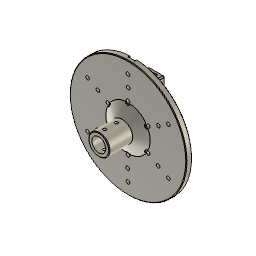
ワインダー量産試作機 (Autodesk Fusion 360 archive; units mm, degrees)
design "ピックアップチャッキ"
Autodesk Fusion 360 part; units mm, degrees
sketch "スケッチ1" plane through (0, 0, 0) normal (0, 0, 1) x (1, 0, 0)
  circle A0 centre (0, 0) radius 50
  dimension "d1" = 100
  constraint coincident A0.centre origin
  measures "d1" diameter of A0
extrude "押し出し1" add sketch "スケッチ1" along normal blind 5 makes body 1
sketch "スケッチ2" plane through (0, 0, 5) normal (0, 0, 1) x (-1, 0, 0)
  circle A0 centre (0, 0) radius 50
  circle A1 centre (0, 0) radius 9
  circle A2 centre (0, 0) radius 6
  dimension "d4" = 18
  dimension "d5" = 12
  constraint concentric A0 A1
  constraint coincident A0.centre A1.centre
  measures "d4" diameter of A1
  measures "d5" diameter of A2
extrude "押し出し2" add sketch "スケッチ2" along normal blind 25 contours A1 bodies 1
sketch "スケッチ3" plane through (0, 0, 0) normal (0, 1, 0) x (1, 0, 0)
  line L0 (9, -5) -> (9, -10)
  line L1 (9, -5) -> (19, -5)
  line L2 (19, -5) -> (9, -10)
  constraint vertical L0
  constraint perpendicular L0 L1
revolve "回転1" add sketch "スケッチ3" angle 360 about axis through (0, 0, 1.75) along (0, 0, 1) bodies 1
chamfer "面取り1" distance 0.5 angle 45 3 edges at (-46.6164, -18.0808, 0) (-46.6164, -18.0808, 5) (8.3909, 3.2545, 30) on bodies 1
sketch "スケッチ4" plane through (0, 0, 0) normal (0, 1, 0) x (1, 0, 0)
  line L0 (0, -30) -> (0, -25)
  line L1 (0, -10) -> (0, -15)
  circle A0 centre (0, -25) radius 1.25
  circle A1 centre (0, -15) radius 1.25
  dimension "d10" = 2.5
  dimension "d11" = 2.5
  constraint vertical L0
  constraint vertical L1
  constraint coincident L0.end A0.centre
  constraint coincident L1.end A1.centre
  measures "d10" diameter of A0
  measures "d11" diameter of A1
extrude "押し出し3" cut sketch "スケッチ4" along normal blind 9 and the other way blind 9 bodies 1
sketch "スケッチ5" plane through (0, 0, 0) normal (0, 0, 1) x (1, 0, 0)
  circle A0 centre (0, -40) radius 1.5
  circle A1 centre (-0.2424, -30) radius 1.5
  circle A2 centre (0, -20) radius 1.5
  point P0 (0, -20)
  point P1 (0, -30)
  point P2 (0, -40)
  dimension "d16" = 3
  dimension "d17" = 3
  dimension "d18" = 3
  constraint coincident P2 A0.centre
  constraint coincident P0 A2.centre
  measures "d16" diameter of A0
  measures "d17" diameter of A1
  measures "d18" diameter of A2
extrude "押し出し4" cut sketch "スケッチ5" along normal blind 6 bodies 1
pattern_circular "C パターン1" count 6 over 360 about axis through (0, 0, 1.75) along (0, 0, 1) of 3 faces at (-1.4095, -39.487, 3.3333) (1.2502, -29.8506, 3.3333) (-1.1427, -19.0283, 3.3333) on bodies 1
sketch "スケッチ6" plane through (0, 0, 0) normal (0, 0, 1) x (1, 0, 0)
  circle A0 centre (0, 0) radius 1.5
  dimension "d23" = 3
  constraint coincident A0.centre origin
  measures "d23" diameter of A0
extrude "押し出し5" cut sketch "スケッチ6" along normal blind 5 bodies 1
sketch "スケッチ7" plane through (0, 0, 5) normal (0, 0, 1) x (-1, 0, 0)
  circle A0 centre (26.1019, 14.7901) radius 1.5
  circle A1 centre (25.8596, -15.2099) radius 1.5
  circle A2 centre (-0.2424, -30) radius 1.5
  circle A3 centre (-26.1019, -14.7901) radius 1.5
  circle A4 centre (-25.8596, 15.2099) radius 1.5
  circle A5 centre (34.641, 20) radius 1.5
  circle A6 centre (34.641, -20) radius 1.5
  circle A7 centre (0, -40) radius 1.5
  circle A8 centre (-34.641, -20) radius 1.5
  circle A9 centre (-34.641, 20) radius 1.5
  arc A10 (16.9721, 8.541) -> (15.8828, 10.4277) centre (17.3205, 10) ccw
  arc A11 (16.9721, -8.541) -> (16.9721, 8.541) centre (0, 0) ccw
  arc A12 (15.8828, -10.4277) -> (16.9721, -8.541) centre (17.3205, -10) ccw
  arc A13 (1.0893, -18.9688) -> (15.8828, -10.4277) centre (0, 0) ccw
  arc A14 (-1.0893, -18.9688) -> (1.0893, -18.9688) centre (0, -20) ccw
  arc A15 (-15.8828, -10.4277) -> (-1.0893, -18.9688) centre (0, 0) ccw
  arc A16 (-16.9721, -8.541) -> (-15.8828, -10.4277) centre (-17.3205, -10) ccw
  arc A17 (-16.9721, 8.541) -> (-16.9721, -8.541) centre (0, 0) ccw
  arc A18 (-15.8828, 10.4277) -> (-16.9721, 8.541) centre (-17.3205, 10) ccw
  arc A19 (-1.0893, 18.9688) -> (-15.8828, 10.4277) centre (0, 0) ccw
  arc A20 (1.0893, 18.9688) -> (-1.0893, 18.9688) centre (0, 20) ccw
  arc A21 (15.8828, 10.4277) -> (1.0893, 18.9688) centre (0, 0) ccw
  circle A22 centre (0.2424, 30) radius 1.5
  circle A23 centre (0, 40) radius 1.5
  circle A24 centre (0, 0) radius 49.5
  circle A25 centre (0, 20) radius 2.5
  circle A26 centre (-17.3205, 10) radius 2.5
  circle A27 centre (-17.3205, -10) radius 2.5
  circle A28 centre (0, -20) radius 2.5
  circle A29 centre (17.3205, -10) radius 2.5
  circle A30 centre (17.3205, 10) radius 2.5
  dimension "d26" = 5
  dimension "d28" = 360
  constraint concentric A20 A25
  measures "d26" diameter of A25
extrude "押し出し6" cut sketch "スケッチ7" along normal blind 1 contours A10 A11 A21 A30 | A11 A12 A13 A29 | A19 A20 A21 A25 | A13 A14 A15 A28 | A17 A18 A19 A26 | A15 A16 A17 A27 picked at (16.0359, 9.1878) picked at (16.0359, -9.1878) picked at (0.2115, 19.7656) picked at (-0.2115, -19.7656) picked at (-16.0331, 9.192) picked at (-17.2117, -9.7715) bodies 1
sketch "スケッチ8" plane through (0, 0, 0) normal (0, 0, -1) x (1, 0, 0)
  circle A0 centre (0, 0) radius 1.5
  circle A1 centre (-26.1019, 14.7901) radius 1.5
  circle A2 centre (-25.8596, -15.2099) radius 1.5
  circle A3 centre (0.2424, -30) radius 1.5
  circle A4 centre (26.1019, -14.7901) radius 1.5
  circle A5 centre (25.8596, 15.2099) radius 1.5
  circle A6 centre (-34.641, 20) radius 1.5
  circle A7 centre (-34.641, -20) radius 1.5
  circle A8 centre (0, -40) radius 1.5
  circle A9 centre (34.641, -20) radius 1.5
  circle A10 centre (34.641, 20) radius 1.5
  circle A11 centre (-17.3205, -10) radius 1.5
  circle A12 centre (17.3205, -10) radius 1.5
  circle A13 centre (0, 0) radius 49.5
  circle A14 centre (0, 40) radius 1.5
  circle A15 centre (-0.2424, 30) radius 1.5
  circle A16 centre (0, 20) radius 1.5
  circle A17 centre (17.3205, 10) radius 1.5
  circle A18 centre (0, -20) radius 1.5
  circle A19 centre (-17.3205, 10) radius 1.5
  line L0 (0, 55) -> (3, 55)
  line L1 (3, 55) -> (-3, 55)
  line L2 (-3, 55) -> (-3, -60.586)
  line L3 (-3, -60.586) -> (3, -60.586)
  line L4 (3, -60.586) -> (3, 55)
  dimension "d31" = 3
  dimension "d32" = 6
  constraint horizontal L0
  constraint horizontal L1
  constraint vertical L2
  constraint horizontal L3
  constraint vertical L4
  measures "d31" distance of L0.start L0.end
  measures "d32" distance of L0.end L1.end
extrude "押し出し7" cut sketch "スケッチ8" against normal blind 2 contours A13 L2 L4 | A13 L0 L1 L2 L4 | A13 L2 L3 L4 bodies 1
sketch "スケッチ9" plane through (0, 0, 5) normal (0, 0, 1) x (-1, 0, 0)
  circle A0 centre (0, 0) radius 1.5
  circle A1 centre (0, 0) radius 6
  line L0 (-2.3, -1.3279) -> (0, -2.6558)
  line L1 (0, -2.6558) -> (2.3, -1.3279)
  line L2 (2.3, -1.3279) -> (2.3, 1.3279)
  line L3 (2.3, 1.3279) -> (0, 2.6558)
  line L4 (0, 2.6558) -> (-2.3, 1.3279)
  line L5 (-2.3, 1.3279) -> (-2.3, -1.3279)
  dimension "d35" = 2.3
  constraint coincident A0.centre A1.centre
  measures "d35" distance of A0.centre L5
extrude "押し出し8" add sketch "スケッチ9" along normal blind 4 contours A1 bodies 1
sketch "スケッチ10" plane through (0, 0, 0) normal (0, 0, 1) x (1, 0, 0)
  line L0 (7, 55) -> (-7, 55)
  line L1 (7, 55) -> (-7, 55)
  line L2 (-7, 55) -> (-7, 115)
  line L3 (-7, 115) -> (7, 115)
  line L4 (7, 115) -> (7, 55)
  constraint horizontal L0
  constraint horizontal L1
  constraint vertical L2
  constraint horizontal L3
  constraint vertical L4
extrude "押し出し9" add sketch "スケッチ10" against normal blind 10 separate body makes body 2
sketch "スケッチ11" plane through (0, 0, -10) normal (0, 0, -1) x (1, 0, 0)
  line L0 (-7, -115) -> (7, -115)
  line L1 (7, -115) -> (7, -55)
  line L2 (7, -55) -> (-7, -55)
  line L3 (-7, -55) -> (-7, -115)
  line L4 (3, -55) -> (-3, -55)
  line L5 (-3, -55) -> (-3, -115)
  line L6 (-3, -115) -> (3, -115)
  line L7 (3, -115) -> (3, -55)
  constraint horizontal L4
  constraint vertical L5
  constraint horizontal L6
  constraint vertical L7
  constraint coincident L0 L5.end
  constraint coincident L2 L4.start
extrude "押し出し10" cut sketch "スケッチ11" against normal blind 7 contours L0 L2 L4 L5 L6 L7 bodies 2
sketch "スケッチ12" plane through (0, 0, -3) normal (0, 0, -1) x (1, 0, 0)
  line L0 (3, -115) -> (3, -55)
  line L1 (3, -55) -> (-3, -55)
  line L2 (-3, -55) -> (-3, -115)
  line L3 (-3, -115) -> (3, -115)
  point P0 (0, -85)
hole "穴1" at (0, 85, -3) direction (0, 0, 1) diameter 3.2 depth 21 tip angle 118 bodies 2
chamfer "面取り2" distance 1 angle 45 10 edges at (7, 85, 0) (-7, 85, 0) (-7, 85, -10) (7, 85, -10) (-7, 115, -5) (7, 115, -5) (0, 115, 0) (0, 55, 0) (7, 55, -5) (-7, 55, -5) on bodies 2
move_body "移動1" bodies 1 to x (1, 0, 0) y (0, 0, 1) z (0, -1, 0) at (0, 0, 0)
move_body "移動2" bodies 2 to x (1, 0, 0) y (0, 0, -1) z (0, 1, 0) at (0, 20, 85)
named bodies: "ピックアップチャッキ", "ピックアップ抑え"
